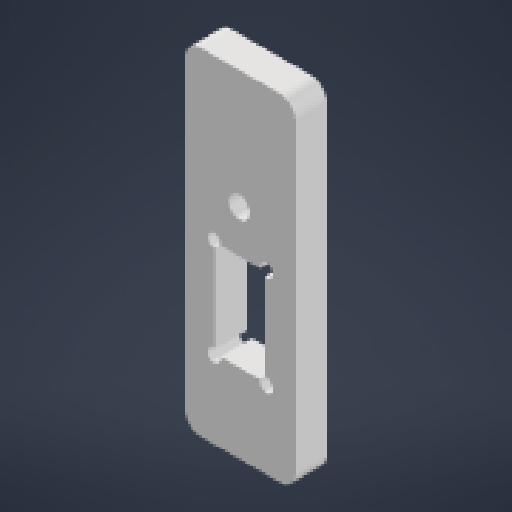
# Autodesk Inventor part: zig2
Saved by Autodesk Inventor 2024.3 (Build 283343000, 343)
## iProperties
Created: 2024-09-11
Part Number: zig2
Material: 일반
Document SubType Name: Modeling
Designer: ASUS
Density: 1 g/cm^3
Appearance: 기본값
Author: ASUS
Autodesk Inventor part; units mm, degrees
ref_plane "YZ Plane" through (0, 0, 0) normal (1, 0, 0) x (0, 1, 0)
ref_plane "XZ Plane" through (0, 0, 0) normal (0, 1, 0) x (-1, 0, 0)
ref_plane "XY Plane" through (0, 0, 0) normal (0, 0, 1) x (1, 0, 0)
ref_plane "작업 평면1" through (0, 0, 0) normal (0, 0, 1) x (1, 0, 0)
sketch "스케치1" plane through (0, 0, 0) normal (0, 0, 1) x (1, 0, 0)
  line L0 (0, -16.5) -> (0, -28.5) projected
  line L1 (0, -28.5) -> (6, -28.5) projected
  line L2 (6, -16.5) -> (6, -28.5) projected
  line L3 (0, -16.5) -> (6, -16.5) projected
  line L4 (6.3, -28.8) -> (-0.3, -28.8)
  line L5 (-0.3, -28.8) -> (-0.3, -16.2)
  line L6 (-0.3, -16.2) -> (6.3, -16.2)
  line L7 (6.3, -16.2) -> (6.3, -28.8)
  circle A0 centre (6.3, -16.2) radius 1.05
  circle A1 centre (6.3, -28.8) radius 1.05
  circle A2 centre (-0.3, -28.8) radius 1.05
  circle A3 centre (-0.3, -16.2) radius 1
  line L8 (0, -15.5) -> (6, -15.5) projected
  line L9 (6, 0) -> (6, -15.5) projected
  line L10 (0, 0) -> (6, 0) projected
  line L11 (0, 0) -> (0, -15.5) projected
  circle A4 centre (2.9, -11) radius 1.35 projected
  line L12 (6, -29.5) -> (0, -29.5) projected
  line L13 (0, -29.5) -> (0, -34.6) projected
  line L14 (0, -34.6) -> (6, -34.6) projected
  line L15 (6, -29.5) -> (6, -34.6) projected
  line L16 (6, 0) -> (0, 0)
  line L17 (0, 0) -> (0, -34.6)
  line L18 (0, -34.6) -> (6, -34.6)
  line L19 (6, -34.6) -> (6, 0)
  line L20 (10, 4) -> (-4, 4)
  line L21 (-4, 4) -> (-4, -38.6)
  line L22 (-4, -38.6) -> (10, -38.6)
  line L23 (10, -38.6) -> (10, 4)
  point P0 (-0.3, -27.75)
  point P1 (-0.3, -17.2)
  point P2 (0.7, -16.2)
  point P3 (5.25, -16.2)
  point P4 (6.3, -17.25)
  point P5 (6.3, -27.75)
  point P6 (5.25, -28.8)
  point P7 (0.75, -28.8)
  dimension "d0" = 0.3
  dimension "d1" = 2.1
  dimension "d2" = 2.1
  dimension "d3" = 2.1
  dimension "d4" = 2
  dimension "d5" = 4
  constraints: 24 end point, 4 centre point, 4 coincident, 4 parallel, 2 perpendicular, 1 horizontal, 6 other
  measures "d0" distance between parallel lines of L2 L7
  measures "d1" diameter of A0
  measures "d2" diameter of A1
  measures "d3" diameter of A2
  measures "d4" diameter of A3
  measures "d5" distance between parallel lines of L19 L23
extrude "돌출1" add sketch "스케치1" along normal blind 4 contours A3 L8 A0 L6 | L11 L10 L9 A0 L8 A3 | L4 A1 L12 A2 | A2 L12 A1 L15 L14 L13 | L23 L22 L21 L20
fillet "모깎기1" radius 2 4 edges at (10, 4, 2) (-4, 4, 2) (10, -38.6, 2) (-4, -38.6, 2)
sketch "스케치2" plane through (0, 0, 0) normal (0, 0, -1) x (-1, 0, 0)
  arc A0 (2, -38.6) -> (4, -36.6) centre (2, -36.6) ccw projected
  line L0 (4, 2) -> (4, -36.6) projected
  arc A1 (4, 2) -> (2, 4) centre (2, 2) ccw projected
  line L1 (-8, 4) -> (2, 4) projected
  arc A2 (-8, 4) -> (-10, 2) centre (-8, 2) ccw projected
  line L2 (-10, -36.6) -> (-10, 2) projected
  arc A3 (-10, -36.6) -> (-8, -38.6) centre (-8, -36.6) ccw projected
  line L3 (2, -38.6) -> (-8, -38.6) projected
  circle A4 centre (-2.9, -11) radius 1.35 projected
  arc A5 (-0.75, -28.8) -> (0.3, -27.75) centre (0.3, -28.8) ccw projected
  line L4 (-5.25, -28.8) -> (-0.75, -28.8) projected
  arc A6 (-6.3, -27.75) -> (-5.25, -28.8) centre (-6.3, -28.8) ccw projected
  line L5 (-6.3, -17.25) -> (-6.3, -27.75) projected
  arc A7 (-5.25, -16.2) -> (-6.3, -17.25) centre (-6.3, -16.2) ccw projected
  line L6 (-0.7, -16.2) -> (-5.25, -16.2) projected
  arc A8 (0.3, -17.2) -> (-0.7, -16.2) centre (0.3, -16.2) ccw projected
  line L7 (0.3, -27.75) -> (0.3, -17.2) projected
  arc A9 (-5.4739, -16.4) -> (-6.1, -17.0261) centre (-6.3, -16.2) ccw
  line L8 (-6.1, -17.0261) -> (-6.1, -27.9739)
  arc A10 (-6.1, -27.9739) -> (-5.4739, -28.6) centre (-6.3, -28.8) ccw
  line L9 (-5.4739, -28.6) -> (-0.5261, -28.6)
  arc A11 (-0.5261, -28.6) -> (0.1, -27.9739) centre (0.3, -28.8) ccw
  line L10 (0.1, -27.9739) -> (0.1, -16.9746)
  arc A12 (0.1, -16.9746) -> (-0.4746, -16.4) centre (0.3, -16.2) ccw
  line L11 (-0.4746, -16.4) -> (-5.4739, -16.4)
  point P0 (0, 0)
  dimension "d9" = 0.2
  constraints: 8 end point, 8 point on circle, 4 centre point, 7 other
  measures "d9" distance between parallel lines of L6 L11
extrude "돌출2" add sketch "스케치2" against normal up to surface (4 mm away) contours L4 A6 L5 A7 L6 A8 L7 A5
sketch "스케치3" plane through (0, 0, 4) normal (0, 0, 1) x (1, 0, 0)
  arc A0 (0.4746, -16.4) -> (-0.1, -16.9746) centre (-0.3, -16.2) ccw projected
  line L0 (5.4739, -16.4) -> (0.4746, -16.4) projected
  arc A1 (6.1, -17.0261) -> (5.4739, -16.4) centre (6.3, -16.2) ccw projected
  line L1 (6.1, -27.9739) -> (6.1, -17.0261) projected
  arc A2 (5.4739, -28.6) -> (6.1, -27.9739) centre (6.3, -28.8) ccw projected
  line L2 (0.5261, -28.6) -> (5.4739, -28.6) projected
  arc A3 (-0.1, -27.9739) -> (0.5261, -28.6) centre (-0.3, -28.8) ccw projected
  line L3 (-0.1, -16.9746) -> (-0.1, -27.9739) projected
  arc A4 (-4, -36.6) -> (-2, -38.6) centre (-2, -36.6) ccw projected
  line L4 (-2, -38.6) -> (8, -38.6) projected
  arc A5 (8, -38.6) -> (10, -36.6) centre (8, -36.6) ccw projected
  line L5 (10, -36.6) -> (10, 2) projected
  arc A6 (10, 2) -> (8, 4) centre (8, 2) ccw projected
  line L6 (8, 4) -> (-2, 4) projected
  arc A7 (-2, 4) -> (-4, 2) centre (-2, 2) ccw projected
  line L7 (-4, 2) -> (-4, -36.6) projected
  circle A8 centre (2.9, -11) radius 1.35 projected
  point P0 (0, 0)
hole "구멍1" at (6.3, -16.2, 4) at (-0.3, -16.2, 4) at (6.3, -28.8, 4) at (-0.3, -28.8, 4) direction (0, 0, -1) diameter 2.1 end through all
